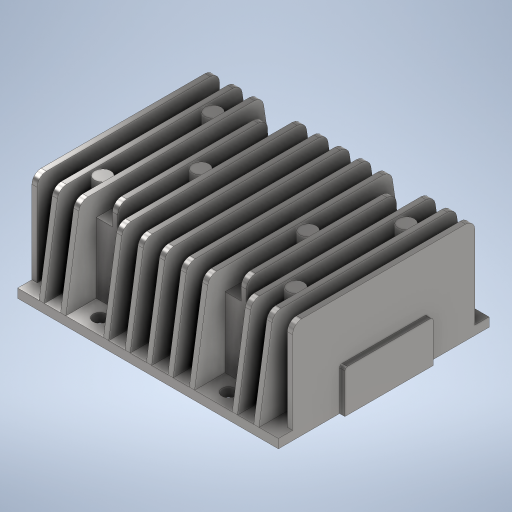
# Autodesk Inventor part: volt-dec-urc
Saved by Autodesk Inventor 2023 (Build 270158000, 158)
## iProperties
Created: 2023-01-08
Part Number: volt-dec-urc
Material: Steel, Alloy
Document SubType Name: Modeling
Designer: t205b
Density: 7.73 g/cm^3
Appearance: Semi-Polished
Mass: 1576.82 g
Surface Area: 517.623 cm^2
Volume: 203.988 cm^3
Author: t205b
Autodesk Inventor part; units mm, degrees
sketch "Sketch2" plane through (0, 0, 0) normal (1, 0, 0) x (0, 1, 0)
  line L0 (0, 40) -> (0, -40)
  line L1 (0, -40) -> (3.4, -40)
  line L2 (3.4, -40) -> (3.4, -34.6)
  line L3 (3.4, -34.6) -> (34.85, -34.6)
  line L4 (38.35, -31.1) -> (38.35, 31.1)
  line L5 (34.85, 34.6) -> (3.4, 34.6)
  line L6 (3.4, 34.6) -> (3.4, 40)
  line L7 (3.4, 40) -> (0, 40)
  line L8 (-7.815, 0) -> (46.8898, 0) projected
  arc A0 (38.35, 31.1) -> (34.85, 34.6) centre (34.85, 31.1) ccw
  arc A1 (34.85, -34.6) -> (38.35, -31.1) centre (34.85, -31.1) ccw
  line L9 (3.4, -34.6) -> (3.4, -28.45)
  line L10 (3.4, -28.45) -> (30, -28.45)
  line L11 (30, -28.45) -> (30, 28.45)
  line L12 (30, 28.45) -> (3.4, 28.45)
  line L13 (3.4, 28.45) -> (3.4, 34.6)
  point P0 (0, 0)
  point P1 (38.35, -34.6)
  point P2 (38.35, 34.6)
  point P3 (19.125, 34.6)
  point P4 (19.125, -34.6)
  dimension "d0" = 38.35
  dimension "d1" = 69.2
  dimension "d4" = 80
  dimension "d5" = 3.4
  dimension "d8" = 3.5
  dimension "d9" = 6.15
  dimension "d10" = 30
  constraints: 26 end point, 8 perpendicular, 7 point on line, 4 point on circle, 4 tangent, 3 vertical, 2 centre point, 2 collinear, 2 midpoint, 2 parallel, 1 equal radius, 1 other
  measures "d0" distance between parallel lines of L0 L4
  measures "d1" distance of point (19.125, 34.6) point (19.125, -34.6)
  measures "d4" distance of L0.start L0.end
  measures "d5" distance of L0.end L1.end
  measures "d8" radius of A0
  measures "d9" distance of L2.end L9.end
  measures "d10" distance between parallel lines of L0 L11
extrude "Extrusion1" add sketch "Sketch2" along normal blind 2
extrude "Extrusion2" add sketch "Sketch2" along normal blind 99 contours L7 L6 L13 L12 L11 L8 L0 | L8 L11 L10 L9 L2 L1 L0
ref_plane "Work Plane1" through (8.15, 0, 0) normal (1, 0, 0) x (0, 0, -1)
sketch "Sketch3" plane through (8.15, 0, 0) normal (1, 0, 0) x (0, 0, -1)
  line L0 (31.1, 38.35) -> (-31.1, 38.35) projected
  line L1 (-34.6, 3.4) -> (-28.45, 3.4) projected
  line L2 (28.45, 3.4) -> (34.6, 3.4) projected
  line L3 (34.6, 3.4) -> (-34.6, 3.4)
  line L4 (-31.1, 38.35) -> (-31.5992, 38.35)
  arc A0 (34.6, 34.85) -> (31.1, 38.35) centre (31.1, 34.85) ccw projected
  line L5 (31.5992, 38.35) -> (31.1, 38.35)
  line L6 (-40, 3.4) -> (-40, 0) projected
  line L7 (-35.0582, 35.3844) -> (-40, 3.4)
  line L8 (40, 3.4) -> (34.6, 3.4) projected
  line L9 (35.0582, 35.3844) -> (40, 3.4)
  arc A1 (-31.5992, 38.35) -> (-35.0582, 35.3844) centre (-31.5992, 34.85) ccw
  arc A2 (35.0582, 35.3844) -> (31.5992, 38.35) centre (31.5992, 34.85) ccw
  line L10 (-40, 3.4) -> (40, 3.4)
  point P0 (0, 0)
  dimension "d16" = 3.5
  constraints: 12 end point, 5 tangent, 4 point on circle, 3 horizontal, 2 centre point, 1 equal radius
  measures "d16" radius of A1
extrude "Extrusion3" add sketch "Sketch3" along normal blind 2
ref_plane "Work Plane2" through (16.3, 0, 0) normal (1, 0, 0) x (0, 0, -1)
sketch "Sketch4" plane through (16.3, 0, 0) normal (1, 0, 0) x (0, 0, -1)
  line L0 (-35.0582, 35.3844) -> (-40, 3.4) projected
  arc A0 (-31.5992, 38.35) -> (-35.0582, 35.3844) centre (-31.5992, 34.85) ccw projected
  line L1 (31.5992, 38.35) -> (-31.5992, 38.35) projected
  line L2 (40, 3.4) -> (35.0582, 35.3844) projected
  arc A1 (35.0582, 35.3844) -> (31.5992, 38.35) centre (31.5992, 34.85) ccw projected
  line L3 (-28.45, 3.4) -> (-40, 3.4) projected
  line L4 (-40, 3.4) -> (40, 3.4)
  point P0 (0, 0)
  constraints: 2 end point, 1 collinear
extrude "Extrusion4" add sketch "Sketch4" along normal blind 2
ref_plane "Work Plane3" through (24.45, 0, 0) normal (1, 0, 0) x (0, 0, -1)
sketch "Sketch5" plane through (24.45, 0, 0) normal (1, 0, 0) x (0, 0, -1)
  line L0 (31.5992, 38.35) -> (-31.5992, 38.35) projected
  line L1 (-28.45, 30) -> (-28.45, 3.4) projected
  line L2 (28.45, 3.4) -> (28.45, 30) projected
  line L3 (-28.45, 30) -> (28.45, 30) projected
  line L4 (-28.45, 30) -> (-28.45, 34.85)
  line L5 (28.45, 30) -> (28.45, 34.85)
  line L6 (31.5992, 38.35) -> (-31.5992, 38.35) projected
  arc A0 (-24.95, 38.35) -> (-28.45, 34.85) centre (-24.95, 34.85) ccw
  arc A1 (28.45, 34.85) -> (24.95, 38.35) centre (24.95, 34.85) ccw
  point P0 (0, 0)
  point P1 (24.95, 38.35)
  point P2 (-24.95, 38.35)
  dimension "d21" = 3.5
  constraints: 4 end point, 4 point on circle, 2 centre point, 2 tangent, 2 vertical, 1 equal radius
  measures "d21" radius of A0
extrude "Extrusion5" add sketch "Sketch5" along normal blind 2
ref_plane "Work Plane4" through (32.6, 0, 0) normal (1, 0, 0) x (0, 0, -1)
sketch "Sketch6" plane through (32.6, 0, 0) normal (1, 0, 0) x (0, 0, -1)
  line L0 (-35.0582, 35.3844) -> (-40, 3.4) projected
  arc A0 (-31.5992, 38.35) -> (-35.0582, 35.3844) centre (-31.5992, 34.85) ccw projected
  line L1 (31.5992, 38.35) -> (-31.5992, 38.35) projected
  line L2 (40, 3.4) -> (35.0582, 35.3844) projected
  arc A1 (35.0582, 35.3844) -> (31.5992, 38.35) centre (31.5992, 34.85) ccw projected
  line L3 (-28.45, 3.4) -> (-40, 3.4) projected
  line L4 (40, 3.4) -> (-40, 3.4)
  point P0 (0, 0)
  constraints: 2 end point
extrude "Extrusion6" add sketch "Sketch6" along normal blind 2
ref_plane "Work Plane5" through (40.75, 0, 0) normal (1, 0, 0) x (0, 0, -1)
sketch "Sketch7" plane through (40.75, 0, 0) normal (1, 0, 0) x (0, 0, -1)
  line L0 (-35.0582, 35.3844) -> (-40, 3.4) projected
  arc A0 (-31.5992, 38.35) -> (-35.0582, 35.3844) centre (-31.5992, 34.85) ccw projected
  line L1 (31.5992, 38.35) -> (-31.5992, 38.35) projected
  arc A1 (35.0582, 35.3844) -> (31.5992, 38.35) centre (31.5992, 34.85) ccw projected
  line L2 (40, 3.4) -> (35.0582, 35.3844) projected
  line L3 (40, 0) -> (40, 3.4) projected
  line L4 (-40, 3.4) -> (40, 3.4)
  point P0 (0, 0)
  constraints: 2 end point
extrude "Extrusion7" add sketch "Sketch7" along normal blind 2
ref_plane "Work Plane6" through (48.9, 0, 0) normal (1, 0, 0) x (0, 0, -1)
sketch "Sketch8" plane through (48.9, 0, 0) normal (1, 0, 0) x (0, 0, -1)
  line L0 (31.5992, 38.35) -> (-31.5992, 38.35) projected
  arc A0 (-31.5992, 38.35) -> (-35.0582, 35.3844) centre (-31.5992, 34.85) ccw projected
  arc A1 (35.0582, 35.3844) -> (31.5992, 38.35) centre (31.5992, 34.85) ccw projected
  line L1 (40, 3.4) -> (35.0582, 35.3844) projected
  line L2 (-35.0582, 35.3844) -> (-40, 3.4) projected
  line L3 (40, 3.4) -> (28.45, 3.4) projected
  line L4 (-40, 3.4) -> (40, 3.4)
  point P0 (0, 0)
  constraints: 2 end point
extrude "Extrusion8" add sketch "Sketch8" along normal blind 2
ref_plane "Work Plane7" through (57.05, 0, 0) normal (1, 0, 0) x (0, 0, -1)
sketch "Sketch9" plane through (57.05, 0, 0) normal (1, 0, 0) x (0, 0, -1)
  line L0 (31.5992, 38.35) -> (-31.5992, 38.35) projected
  line L1 (-35.0582, 35.3844) -> (-40, 3.4) projected
  arc A0 (-31.5992, 38.35) -> (-35.0582, 35.3844) centre (-31.5992, 34.85) ccw projected
  arc A1 (35.0582, 35.3844) -> (31.5992, 38.35) centre (31.5992, 34.85) ccw projected
  line L2 (40, 3.4) -> (35.0582, 35.3844) projected
  line L3 (-34.6, 3.4) -> (-40, 3.4) projected
  line L4 (-40, 3.4) -> (40, 3.4)
  point P0 (0, 0)
  constraints: 2 end point
extrude "Extrusion9" add sketch "Sketch9" along normal blind 2
ref_plane "Work Plane8" through (65.2, 0, 0) normal (1, 0, 0) x (0, 0, -1)
sketch "Sketch10" plane through (65.2, 0, 0) normal (1, 0, 0) x (0, 0, -1)
  line L0 (31.5992, 38.35) -> (-31.5992, 38.35) projected
  line L1 (-35.0582, 35.3844) -> (-40, 3.4) projected
  arc A0 (-31.5992, 38.35) -> (-35.0582, 35.3844) centre (-31.5992, 34.85) ccw projected
  arc A1 (35.0582, 35.3844) -> (31.5992, 38.35) centre (31.5992, 34.85) ccw projected
  line L2 (40, 3.4) -> (35.0582, 35.3844) projected
  line L3 (-28.45, 3.4) -> (-40, 3.4) projected
  line L4 (-40, 3.4) -> (40, 3.4)
  point P0 (0, 0)
  constraints: 2 end point, 1 horizontal
extrude "Extrusion10" add sketch "Sketch10" along normal blind 2
ref_plane "Work Plane9" through (73.35, 0, 0) normal (1, 0, 0) x (0, 0, -1)
sketch "Sketch11" plane through (73.35, 0, 0) normal (1, 0, 0) x (0, 0, -1)
  line L0 (28.45, 30) -> (-28.45, 30) projected
  line L1 (28.45, 30) -> (28.45, 34.85) projected
  arc A0 (28.45, 34.85) -> (24.95, 38.35) centre (24.95, 34.85) ccw projected
  line L2 (24.95, 38.35) -> (-24.95, 38.35) projected
  arc A1 (-24.95, 38.35) -> (-28.45, 34.85) centre (-24.95, 34.85) ccw projected
  line L3 (-28.45, 34.85) -> (-28.45, 30) projected
  point P0 (0, 0)
extrude "Extrusion11" add sketch "Sketch11" along normal blind 2
ref_plane "Work Plane10" through (81.5, 0, 0) normal (1, 0, 0) x (0, 0, -1)
sketch "Sketch12" plane through (81.5, 0, 0) normal (1, 0, 0) x (0, 0, -1)
  line L0 (28.45, 3.4) -> (28.45, 30) projected
  line L1 (40, 3.4) -> (28.45, 3.4) projected
  line L2 (40, 3.4) -> (35.0582, 35.3844) projected
  arc A0 (35.0582, 35.3844) -> (31.5992, 38.35) centre (31.5992, 34.85) ccw projected
  line L3 (31.5992, 38.35) -> (-31.5992, 38.35) projected
  arc A1 (-31.5992, 38.35) -> (-35.0582, 35.3844) centre (-31.5992, 34.85) ccw projected
  line L4 (-35.0582, 35.3844) -> (-40, 3.4) projected
  line L5 (-28.45, 3.4) -> (-40, 3.4) projected
  line L6 (-28.45, 30) -> (-28.45, 3.4) projected
  line L7 (28.45, 30) -> (-28.45, 30) projected
  point P0 (0, 0)
extrude "Extrusion12" add sketch "Sketch12" along normal blind 2
ref_plane "Work Plane11" through (89.65, 0, 0) normal (1, 0, 0) x (0, 0, -1)
sketch "Sketch13" plane through (89.65, 0, 0) normal (1, 0, 0) x (0, 0, -1)
  arc A0 (35.0582, 35.3844) -> (31.5992, 38.35) centre (31.5992, 34.85) ccw projected
  line L0 (31.5992, 38.35) -> (-31.5992, 38.35) projected
  arc A1 (-31.5992, 38.35) -> (-35.0582, 35.3844) centre (-31.5992, 34.85) ccw projected
  line L1 (-35.0582, 35.3844) -> (-40, 3.4) projected
  line L2 (-28.45, 3.4) -> (-40, 3.4) projected
  line L3 (-28.45, 30) -> (-28.45, 3.4) projected
  line L4 (28.45, 30) -> (-28.45, 30) projected
  line L5 (28.45, 3.4) -> (28.45, 30) projected
  line L6 (40, 3.4) -> (28.45, 3.4) projected
  line L7 (40, 3.4) -> (35.0582, 35.3844) projected
  point P0 (0, 0)
extrude "Extrusion13" add sketch "Sketch13" along normal blind 2
sketch "Sketch14" plane through (99, 0, 0) normal (1, 0, 0) x (0, 0, -1)
  line L0 (28.45, 3.4) -> (34.6, 3.4) projected
  line L1 (34.6, 3.4) -> (34.6, 34.85) projected
  arc A0 (34.6, 34.85) -> (31.1, 38.35) centre (31.1, 34.85) ccw projected
  line L2 (31.1, 38.35) -> (-31.1, 38.35) projected
  arc A1 (-31.1, 38.35) -> (-34.6, 34.85) centre (-31.1, 34.85) ccw projected
  line L3 (-34.6, 34.85) -> (-34.6, 3.4) projected
  line L4 (-34.6, 3.4) -> (-28.45, 3.4) projected
  line L5 (-28.45, 3.4) -> (-28.45, 30) projected
  line L6 (-28.45, 30) -> (28.45, 30) projected
  line L7 (28.45, 30) -> (28.45, 3.4) projected
  point P0 (0, 0)
extrude "Extrusion14" add sketch "Sketch14" against normal blind 2
sketch "Sketch15" plane through (67.2, 3.4, 40) normal (0, 1, 0) x (1, 0, 0)
  circle A0 centre (7.15, 5.775) radius 2.6
  circle A1 centre (7.15, 74.225) radius 2.6
  circle A2 centre (-41.75, 74.225) radius 2.6
  circle A3 centre (-41.75, 5.775) radius 2.6
  line L0 (-42.75, 96) -> (-42.75, -16) projected
  line L1 (6.15, 96) -> (6.15, -16) projected
  line L2 (0, 68.45) -> (6.15, 68.45) projected
  line L3 (14.3, 68.45) -> (14.3, 80) projected
  line L4 (0, 80) -> (14.3, 80) projected
  line L5 (0, 80) -> (0, 68.45) projected
  line L6 (0, 68.45) -> (14.3, 68.45) projected
  line L7 (0, 0) -> (14.3, 0) projected
  line L8 (-48.9, 0) -> (-34.6, 0) projected
  line L9 (-48.9, 80) -> (-34.6, 80) projected
  point P0 (-67.2, 40)
  dimension "d50" = 5.2
  dimension "d51" = 5.2
  dimension "d52" = 5.2
  dimension "d53" = 5.2
  dimension "d54" = 1
  dimension "d55" = 1
  dimension "d56" = 1
  dimension "d57" = 1
  dimension "d58" = 11.55
  dimension "d59" = 5.775
  dimension "d60" = 5.775
  dimension "d61" = 5.775
  dimension "d62" = 5.775
  constraints: 4 centre point
  measures "d50" diameter of A0
  measures "d51" diameter of A1
  measures "d52" diameter of A2
  measures "d53" diameter of A3
  measures "d54" distance from line of A3.centre L0
  measures "d55" distance from line of L0 A2.centre
  measures "d56" distance from line of L1 A0.centre
  measures "d57" distance from line of L1 A1.centre
  measures "d58" distance of L4.start L5.end
  measures "d59" distance from line of A1.centre L4
  measures "d60" distance from line of L7 A0.centre
  measures "d61" distance from line of L8 A3.centre
  measures "d62" distance from line of A2.centre L9
extrude "Extrusion15" cut sketch "Sketch15" against normal through all contours A0 L1 | L1 A0 | L1 A1 | A1 L1 | A2 L0 | A3 L0 | L0 A3 | L0 A2
sketch "Sketch16" plane through (26.45, 30, 28.45) normal (0, 1, 0) x (1, 0, 0)
  circle A0 centre (3.075, 28.45) radius 3.075
  circle A1 centre (43.825, 28.45) radius 3.075
  circle A2 centre (-13.225, 49.4) radius 3.075
  circle A3 centre (-13.225, 7.5) radius 3.075
  circle A4 centre (60.125, 49.4) radius 3.075
  circle A5 centre (60.125, 7.5) radius 3.075
  line L0 (38.75, 84.45) -> (38.75, -27.55) projected
  line L1 (0, 56.9) -> (6.15, 56.9) projected
  line L2 (0, 0) -> (6.15, 0) projected
  line L3 (0, 53.4) -> (0, 3.5) projected
  line L4 (46.9, 84.45) -> (46.9, -27.55) projected
  line L5 (-10.15, 84.45) -> (-10.15, -27.55) projected
  line L6 (63.2, 84.45) -> (63.2, -27.55) projected
  line L7 (-16.3, 56.9) -> (-10.15, 56.9) projected
  line L8 (57.05, 56.9) -> (63.2, 56.9) projected
  line L9 (-16.3, 0) -> (-10.15, 0) projected
  line L10 (57.05, 0) -> (63.2, 0) projected
  point P0 (-26.45, 28.45)
  point P1 (3.075, 0)
  point P2 (3.075, 56.9)
  point P3 (-13.225, 56.9)
  point P4 (60.125, 56.9)
  point P5 (-13.225, 0)
  dimension "d65" = 6.15
  dimension "d66" = 6.15
  dimension "d67" = 6.15
  dimension "d68" = 6.15
  dimension "d69" = 6.15
  dimension "d70" = 6.15
  dimension "d71" = 56.9
  dimension "d72" = 28.45
  dimension "d73" = 28.45
  dimension "d74" = 3.075
  dimension "d75" = 3.075
  dimension "d76" = 3.075
  dimension "d77" = 3.075
  dimension "d78" = 3.075
  dimension "d79" = 3.075
  dimension "d80" = 7.5
  dimension "d81" = 7.5
  dimension "d82" = 7.5
  dimension "d83" = 7.5
  constraints: 6 centre point, 5 midpoint
  measures "d65" diameter of A0
  measures "d66" diameter of A1
  measures "d67" diameter of A2
  measures "d68" diameter of A3
  measures "d69" diameter of A4
  measures "d70" diameter of A5
  measures "d71" distance of point (3.075, 0) point (3.075, 56.9)
  measures "d72" distance from line of L1 A0.centre
  measures "d73" distance from line of A1.centre L1
  measures "d74" distance from line of A0.centre L3
  measures "d75" distance from line of A1.centre L4
  measures "d76" distance from line of A3.centre L5
  measures "d77" distance from line of A2.centre L5
  measures "d78" distance from line of A5.centre L6
  measures "d79" distance from line of A4.centre L6
  measures "d80" distance of point (-13.225, 56.9) A2.centre
  measures "d81" distance of point (60.125, 56.9) A4.centre
  measures "d82" distance of A3.centre point (-13.225, 0)
  measures "d83" distance from line of A5.centre L10
extrude "Extrusion16" add sketch "Sketch16" along normal blind 7.5
sketch "Sketch17" plane through (99, 0, 0) normal (1, 0, 0) x (0, 0, -1)
  line L0 (-40, 0) -> (40, 0) projected
  line L1 (-16.75, 16) -> (16.75, 16)
  line L2 (16.75, 16) -> (16.75, 0)
  line L3 (16.75, 0) -> (-16.75, 0)
  line L4 (-16.75, 0) -> (-16.75, 16)
  line L5 (-34.6, 34.85) -> (-34.6, 3.4) projected
  line L6 (34.6, 3.4) -> (34.6, 34.85) projected
  point P0 (0, 0)
  point P1 (-16.75, 8)
  dimension "d86" = 16
  dimension "d87" = 33.5
  dimension "d88" = 17.85
  dimension "d89" = 69.2
  constraints: 8 end point, 2 parallel, 1 horizontal, 1 midpoint, 1 perpendicular, 1 point on line
  measures "d86" distance between parallel lines of L1 L0
  measures "d87" distance from line of point (-16.75, 8) L2
  measures "d88" distance between parallel lines of L4 L5
  measures "d89" distance between parallel lines of L6 L5
extrude "Extrusion17" add sketch "Sketch17" along normal blind 2
fillet "Fillet1" radius 1 2 edges at (100, 16, -16.75) (100, 16, 16.75)
equation "\"d9\" = spacing"
equation "\"d59\" = 0.5 * d58"
equation "\"d60\" = 0.5 * d58"
equation "\"d61\" = 0.5 * d58"
equation "\"d62\" = 0.5 * d58"
equation "\"d65\" = spacing"
equation "\"d66\" = spacing"
equation "\"d67\" = spacing"
equation "\"d68\" = spacing"
equation "\"d69\" = spacing"
equation "\"d70\" = spacing"
equation "\"d72\" = 0.5 * d71"
equation "\"d73\" = 0.5 * d71"
equation "\"d74\" = 0.5 * spacing"
equation "\"d75\" = 0.5 * spacing"
equation "\"d76\" = 0.5 * spacing"
equation "\"d77\" = 0.5 * spacing"
equation "\"d78\" = 0.5 * spacing"
equation "\"d79\" = 0.5 * spacing"
equation "\"d88\" = 0.5 * d89 - 0.5 * d87"
equation "\"spacing\" = 6.15"
body "Solid1"
